Autodesk Inventor part; units mm, degrees
(part 3 of 3)
  line L490 (25.75, 63.25) -> (51.25, 63.25)
  line L491 (51.25, 63.25) -> (51.25, 73.75)
  line L492 (51.25, 73.75) -> (25.75, 73.75)
  line L493 (25.75, 73.75) -> (25.75, 63.25)
  line L494 (25.75, 78.25) -> (51.25, 78.25)
  line L495 (51.25, 78.25) -> (51.25, 88.75)
  line L496 (51.25, 88.75) -> (25.75, 88.75)
  line L497 (25.75, 88.75) -> (25.75, 78.25)
  line L498 (25.75, 93.25) -> (51.25, 93.25)
  line L499 (51.25, 93.25) -> (51.25, 103.75)
  line L500 (51.25, 103.75) -> (25.75, 103.75)
  line L501 (25.75, 103.75) -> (25.75, 93.25)
  line L502 (25.75, 108.25) -> (51.25, 108.25)
  line L503 (51.25, 108.25) -> (51.25, 118.75)
  line L504 (51.25, 118.75) -> (25.75, 118.75)
  line L505 (25.75, 118.75) -> (25.75, 108.25)
  line L506 (10.75, -86.75) -> (21.25, -86.75)
  line L507 (21.25, -86.75) -> (21.25, -68.75)
  line L508 (21.25, -68.75) -> (10.75, -68.75)
  line L509 (10.75, -68.75) -> (10.75, -86.75)
  line L510 (10.75, -46.25) -> (21.25, -46.25)
  line L511 (21.25, -46.25) -> (21.25, -64.25)
  line L512 (21.25, -64.25) -> (10.75, -64.25)
  line L513 (10.75, -64.25) -> (10.75, -46.25)
  line L514 (10.75, -41.75) -> (21.25, -41.75)
  line L515 (21.25, -41.75) -> (21.25, -23.75)
  line L516 (21.25, -23.75) -> (10.75, -23.75)
  line L517 (10.75, -23.75) -> (10.75, -41.75)
  line L518 (10.75, -19.25) -> (21.25, -19.25)
  line L519 (21.25, -19.25) -> (21.25, -8.75)
  line L520 (21.25, -8.75) -> (10.75, -8.75)
  line L521 (10.75, -8.75) -> (10.75, -19.25)
  line L522 (10.75, 13.75) -> (21.25, 13.75)
  line L523 (21.25, 13.75) -> (21.25, -4.25)
  line L524 (21.25, -4.25) -> (10.75, -4.25)
  line L525 (10.75, -4.25) -> (10.75, 13.75)
  line L526 (10.75, 18.25) -> (21.25, 18.25)
  line L527 (21.25, 18.25) -> (21.25, 36.25)
  line L528 (21.25, 36.25) -> (10.75, 36.25)
  line L529 (10.75, 36.25) -> (10.75, 18.25)
  line L530 (10.75, 58.75) -> (21.25, 58.75)
  line L531 (21.25, 58.75) -> (21.25, 40.75)
  line L532 (21.25, 40.75) -> (10.75, 40.75)
  line L533 (10.75, 40.75) -> (10.75, 58.75)
  line L534 (10.75, 63.25) -> (21.25, 63.25)
  line L535 (21.25, 63.25) -> (21.25, 81.25)
  line L536 (21.25, 81.25) -> (10.75, 81.25)
  line L537 (10.75, 81.25) -> (10.75, 63.25)
  line L538 (10.75, 118.75) -> (21.25, 118.75)
  line L539 (21.25, 118.75) -> (21.25, 100.75)
  line L540 (21.25, 100.75) -> (10.75, 100.75)
  line L541 (10.75, 100.75) -> (10.75, 118.75)
  line L542 (10.75, 85.75) -> (21.25, 85.75)
  line L543 (21.25, 85.75) -> (21.25, 96.25)
  line L544 (21.25, 96.25) -> (10.75, 96.25)
  line L545 (10.75, 96.25) -> (10.75, 85.75)
  point P0 (0, 0)
  point P1 (10.75, -64.25)
  point P2 (21.25, -53.75)
  point P3 (21.25, -49.25)
  point P4 (21.25, -8.75)
  point P5 (21.25, 36.25)
  point P6 (10.75, 40.75)
  point P7 (21.25, 51.25)
  point P8 (21.25, 55.75)
  point P9 (21.25, 96.25)
  dimension "d223" = 0.25
  dimension "d224" = 10.5
  dimension "d225" = 10.5
  dimension "d226" = 0.25
  dimension "d229" = 15
  dimension "d232" = 15
  dimension "d283" = 10.5
  dimension "d284" = 18
  dimension "d285" = 18
  dimension "d286" = 18
  dimension "d287" = 10.5
  dimension "d288" = 4.5
  dimension "d289" = 18
  dimension "d290" = 18
  dimension "d291" = 18
  dimension "d292" = 18
  dimension "d293" = 18
  dimension "d294" = 10.5
  dimension "d295" = 4.5
  constraints: 1088 end point, 50 parallel, 26 horizontal, 25 perpendicular, 21 point on line, 2 collinear, 1 vertical, 886 other
  measures "d223" distance between parallel lines of L4 L0
  measures "d224" distance of L0.start L0.end
  measures "d225" distance of L0.end L1.end
  measures "d226" distance between parallel lines of L5 L3
  measures "d229" distance of L0.start L6.start
  measures "d232" distance of L0.start L66.start
  measures "d283" distance of L508.end L507.end
  measures "d284" distance of L507.end L506.end
  measures "d285" distance of L510.end L511.end
  measures "d286" distance of L514.end L515.end
  measures "d287" distance of L518.end L519.end
  measures "d288" distance between parallel lines of L516 L518
  measures "d289" distance of L522.end L523.end
  measures "d290" distance of L526.end L527.end
  measures "d291" distance of L530.end L531.end
  measures "d292" distance of L534.end L535.end
  measures "d293" distance of L538.end L539.end
  measures "d294" distance of L542.end L543.end
  measures "d295" distance between parallel lines of L536 L542
extrude "Extrusion8" add sketch "Sketch21" along normal blind 1 contours L0 L1 L2 L3 | L6 L7 L8 L9 | L66 L67 L68 L69 | L70 L71 L72 L73 | L130 L131 L132 L133 | L134 L135 L136 L137 | L162 L163 L164 L165 | L166 L167 L168 L169 | L170 L171 L172 L173 | L174 L175 L176 L177 | L178 L179 L180 L181 | L182 L183 L184 L185 | L186 L187 L188 L189 | L190 L191 L192 L193 | L194 L195 L196 L197 | L198 L199 L200 L201 | L226 L227 L228 L229 | L230 L231 L232 L233 | L234 L235 L236 L237 | L238 L239 L240 L241 | L242 L243 L244 L245 | L246 L247 L248 L249 | L250 L251 L252 L253 | L254 L255 L256 L257 | L258 L259 L260 L261 | L262 L263 L264 L265 | L266 L267 L268 L269 | L268 L509 L270 L507 | L270 L271 L508 L273 | L512 L271 L272 L273 | L272 L513 L274 L511 | L274 L275 L276 L277 | L278 L279 L280 L281 | L280 L517 L282 L515 | L282 L283 L516 L285 | L518 L283 L284 L285 | L284 L521 L286 L519 | L286 L287 L520 L289 | L524 L287 L288 L289 | L288 L525 L290 L523 | L290 L291 L292 L293 | L294 L295 L296 L297 | L296 L529 L298 L527 | L298 L299 L528 L301 | L532 L299 L300 L301 | L300 L533 L302 L531 | L302 L303 L304 L305 | L306 L307 L308 L309 | L308 L537 L310 L535 | L310 L311 L536 L313 | L542 L311 L312 L313 | L312 L545 L314 L543 | L314 L315 L544 L317 | L540 L315 L316 L317 | L316 L541 L318 L539 | L318 L319 L320 L321 | L322 L323 L324 L325 | L326 L327 L328 L329 | L330 L331 L332 L333 | L333 L452 L395 L450 | L395 L396 L397 L394 | L334 L335 L336 L337 | L337 L456 L399 L454 | L399 L400 L401 L398 | L338 L339 L340 L341 | L341 L460 L403 L458 | L403 L404 L405 L402 | L342 L343 L344 L345 | L345 L464 L407 L462 | L407 L408 L409 L406 | L346 L347 L348 L349 | L349 L468 L411 L466 | L411 L412 L413 L410 | L350 L351 L352 L353 | L353 L472 L415 L470 | L415 L416 L417 L414 | L354 L355 L356 L357 | L357 L476 L419 L474 | L419 L420 L421 L418 | L358 L359 L360 L361 | L361 L480 L423 L478 | L423 L424 L425 L422 | L362 L363 L364 L365 | L365 L484 L427 L482 | L427 L428 L429 L426 | L366 L367 L368 L369 | L369 L488 L431 L486 | L431 L432 L433 L430 | L370 L371 L372 L373 | L373 L492 L435 L490 | L435 L436 L437 L434 | L374 L375 L376 L377 | L377 L496 L439 L494 | L439 L440 L441 L438 | L378 L379 L380 L381 | L381 L500 L443 L498 | L443 L444 L445 L442 | L382 L383 L384 L385 | L385 L504 L447 L502 | L447 L448 L449 L446 | L386 L387 L388 L389 | L390 L391 L392 L393
body "Solid1"
